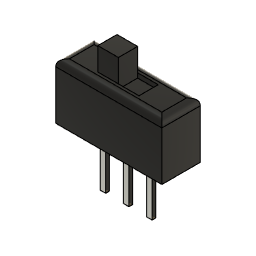
dropEgg_02 v12 (Autodesk Fusion 360 archive; units mm, degrees)
design "Switch"
Autodesk Fusion 360 part; units mm, degrees
sketch "Sketch1" plane through (0, 0, 0) normal (0, 0, 1) x (1, 0, 0)
  line L0 (5.8, -2.1) -> (-5.8, -2.1)
  line L1 (-5.8, -2.1) -> (-5.8, 2.1)
  line L2 (-5.8, 2.1) -> (5.8, 2.1)
  line L3 (5.8, 2.1) -> (5.8, -2.1)
  line L4 (5.8, -2.1) -> (-5.8, 2.1) construction
  line L5 (-5.8, -2.1) -> (5.8, 2.1) construction
  dimension "d1" = 11.6
  dimension "d2" = 4.2
  constraint horizontal L0
  constraint perpendicular L0 L1
  constraint parallel L0 L2
  constraint parallel L1 L3
  constraint coincident L4 origin
  constraint coincident L5 origin
  measures "d1" distance of L1.end L2.end
  measures "d2" distance of L0.end L1.end
extrude "Extrude1" add sketch "Sketch1" along normal blind 6.1
sketch "Sketch2" plane through (0, 0, 6.1) normal (0, 0, 1) x (-1, 0, 0)
  line L0 (-5.8, -2.1) -> (5.8, -2.1)
  line L1 (5.8, -2.1) -> (5.8, 2.1)
  line L2 (5.8, 2.1) -> (-5.8, 2.1)
  line L3 (-5.8, 2.1) -> (-5.8, -2.1)
  line L4 (-2.25, 1.05) -> (2.25, 1.05)
  line L5 (2.25, 1.05) -> (2.25, -1.05)
  line L6 (2.25, -1.05) -> (-2.25, -1.05)
  line L7 (-2.25, -1.05) -> (-2.25, 1.05)
  line L8 (-2.25, 1.05) -> (2.25, -1.05) construction
  line L9 (2.25, 1.05) -> (-2.25, -1.05) construction
  line L10 (0, -1.05) -> (0, 1.05)
  dimension "d5" = 4.5
  dimension "d6" = 2.1
  constraint horizontal L4
  constraint perpendicular L4 L5
  constraint parallel L4 L6
  constraint parallel L5 L7
  constraint coincident L8 origin
  constraint coincident L9 origin
  constraint midpoint L6 L10.start
  constraint midpoint L4 L10.end
  measures "d5" distance of L5.end L6.end
  measures "d6" distance of L4.end L5.end
extrude "Extrude2" add sketch "Sketch2" along normal blind 2.5 contours L4 L5 L6 L10
extrude "Extrude3" cut sketch "Sketch2" against normal blind 0.5 contours L4 L6 L7 L10
sketch "Sketch3" plane through (0, 0, 0) normal (0, 0, -1) x (1, 0, 0)
  line L0 (-5.8, -2.1) -> (5.8, -2.1)
  line L1 (5.8, -2.1) -> (5.8, 2.1)
  line L2 (5.8, 2.1) -> (-5.8, 2.1)
  line L3 (-5.8, 2.1) -> (-5.8, -2.1)
  line L4 (0.3, -0.2) -> (-0.3, -0.2)
  line L5 (-0.3, -0.2) -> (-0.3, 0.2)
  line L6 (-0.3, 0.2) -> (0.3, 0.2)
  line L7 (0.3, 0.2) -> (0.3, -0.2)
  line L8 (0.3, -0.2) -> (-0.3, 0.2) construction
  line L9 (-0.3, -0.2) -> (0.3, 0.2) construction
  dimension "d11" = 0.6
  dimension "d12" = 0.4
  constraint horizontal L4
  constraint perpendicular L4 L5
  constraint parallel L4 L6
  constraint parallel L5 L7
  constraint coincident L8 origin
  constraint coincident L9 origin
  measures "d11" distance of L5.end L6.end
  measures "d12" distance of L4.end L5.end
extrude "Extrude4" add sketch "Sketch3" along normal blind 5.8 contours L4 L5 L6 L7
pattern_linear "R-Pattern1" count 3 spacing 2.54 along (-1, 0, 0) both ways of "Extrude4"
fillet "Fillet1" radius 0.75 tangency weight 1.40143 4 edges at (-5.8, 0, 6.1) (5.8, 0, 6.1) (0, -2.1, 6.1) (0, 2.1, 6.1)

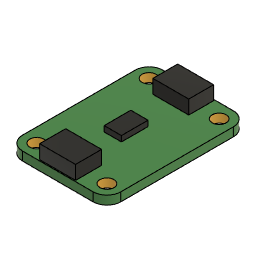
design "ADXL575"
Autodesk Fusion 360 part; units mm, degrees
sketch "Sketch1" plane through (0, 0, 0) normal (0, 0, 1) x (1, 0, 0)
  line L0 (8.89, -12.7) -> (-8.89, -12.7)
  line L1 (-8.89, -12.7) -> (-8.89, 12.7)
  line L2 (-8.89, 12.7) -> (8.89, 12.7)
  line L3 (8.89, 12.7) -> (8.89, -12.7)
  line L4 (8.89, -12.7) -> (-8.89, 12.7) construction
  line L5 (-8.89, -12.7) -> (8.89, 12.7) construction
  line L6 (6.35, -10.16) -> (-6.35, -10.16) construction
  line L7 (-6.35, -10.16) -> (-6.35, 10.16) construction
  line L8 (-6.35, 10.16) -> (6.35, 10.16) construction
  line L9 (6.35, 10.16) -> (6.35, -10.16) construction
  line L10 (6.35, -10.16) -> (-6.35, 10.16) construction
  line L11 (-6.35, -10.16) -> (6.35, 10.16) construction
  circle A0 centre (-6.35, 10.16) radius 1.27
  circle A1 centre (6.35, 10.16) radius 1.27
  circle A2 centre (-6.35, -10.16) radius 1.27
  circle A3 centre (6.35, -10.16) radius 1.27
  dimension "d1" = 17.78
  dimension "d2" = 25.4
  dimension "d3" = 12.7
  dimension "d4" = 20.32
  dimension "d5" = 2.54
  dimension "d6" = 2.54
  dimension "d7" = 2.54
  dimension "d8" = 2.54
  constraint horizontal L0
  constraint perpendicular L0 L1
  constraint parallel L0 L2
  constraint parallel L1 L3
  constraint coincident L4 origin
  constraint coincident L5 origin
  constraint horizontal L6
  constraint perpendicular L6 L7
  constraint parallel L6 L8
  constraint parallel L7 L9
  constraint coincident L10 origin
  constraint coincident L11 origin
  constraint coincident L7.end L8.start
  constraint coincident L8.end L9.start
  constraint coincident L6.end L7.start
  constraint coincident L6.start L9.end
  measures "d1" distance of L1.end L2.end
  measures "d2" distance of L0.end L1.end
  measures "d3" distance of L7.end L8.end
  measures "d4" distance of L6.end L7.end
  measures "d5" diameter of A0
  measures "d6" diameter of A1
  measures "d7" diameter of A2
  measures "d8" diameter of A3
extrude "Extrude1" add sketch "Sketch1" along normal blind 1.57
fillet "Fillet1" radius 2.5 4 edges at (-8.89, -12.7, 0.785) (8.89, -12.7, 0.785) (8.89, 12.7, 0.785) (-8.89, 12.7, 0.785)
sketch "Sketch2" plane through (0, 0, 1.57) normal (0, 0, 1) x (-1, 0, 0)
  arc A0 (6.39, -12.7) -> (8.89, -10.2) centre (6.39, -10.2) ccw
  line L0 (8.89, -10.2) -> (8.89, 10.2)
  arc A1 (8.89, 10.2) -> (6.39, 12.7) centre (6.39, 10.2) ccw
  line L1 (6.39, 12.7) -> (-6.39, 12.7)
  arc A2 (-6.39, 12.7) -> (-8.89, 10.2) centre (-6.39, 10.2) ccw
  line L2 (-8.89, 10.2) -> (-8.89, -10.2)
  arc A3 (-8.89, -10.2) -> (-6.39, -12.7) centre (-6.39, -10.2) ccw
  line L3 (-6.39, -12.7) -> (6.39, -12.7)
  circle A4 centre (6.35, -10.16) radius 1.27
  circle A5 centre (6.35, 10.16) radius 1.27
  circle A6 centre (-6.35, -10.16) radius 1.27
  circle A7 centre (-6.35, 10.16) radius 1.27
  line L4 (2, -2.5) -> (-1.1251, -2.5)
  line L5 (-1.1251, -2.5) -> (-1.1251, 2.3163)
  line L6 (-1.1251, 2.3163) -> (2, 2.3163)
  line L7 (2, 2.3163) -> (2, -2.5)
  line L8 (3.5, -12.5) -> (-3, -12.5)
  line L9 (-3, -12.5) -> (-3, -8)
  line L10 (-3, -8) -> (3.5, -8)
  line L11 (3.5, -8) -> (3.5, -12.5)
  line L12 (3.5, 12.5) -> (-3, 12.5)
  line L13 (-3, 12.5) -> (-3, 7.7871)
  line L14 (-3, 7.7871) -> (3.5, 7.7871)
  line L15 (3.5, 7.7871) -> (3.5, 12.5)
  constraint horizontal L4
  constraint vertical L5
  constraint horizontal L6
  constraint vertical L7
  constraint horizontal L8
  constraint vertical L9
  constraint horizontal L10
  constraint vertical L11
  constraint horizontal L12
  constraint vertical L13
  constraint horizontal L14
  constraint vertical L15
extrude "Extrude2" add sketch "Sketch2" along normal blind 2.5 contours L8 L9 L10 L11 | L12 L13 L14 L15
extrude "Extrude3" add sketch "Sketch2" along normal blind 1 contours L4 L5 L6 L7
equation "d1 = ( 0.7 * 25.4 ) * 1 mm"
equation "d3 = ( 0.5 * 25.4 ) * 1 mm"
equation "d4 = ( 0.8 * 25.4 ) * 1 mm"

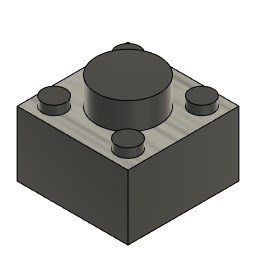
design "microswitch"
Autodesk Fusion 360 part; units mm, degrees
sketch "Sketch1" plane through (0, 0, 0) normal (0, 0, 1) x (1, 0, 0)
  line L0 (3.075, -3.075) -> (-3.075, -3.075)
  line L1 (-3.075, -3.075) -> (-3.075, 3.075)
  line L2 (-3.075, 3.075) -> (3.075, 3.075)
  line L3 (3.075, 3.075) -> (3.075, -3.075)
  line L4 (3.075, -3.075) -> (-3.075, 3.075) construction
  line L5 (-3.075, -3.075) -> (3.075, 3.075) construction
  circle A0 centre (0, 0) radius 1.75
  line L6 (2.05, 2.05) -> (-2.05, 2.05) construction
  line L7 (-2.05, 2.05) -> (-2.05, -2.05) construction
  line L8 (-2.05, -2.05) -> (2.05, -2.05) construction
  line L9 (2.05, -2.05) -> (2.05, 2.05) construction
  line L10 (2.05, 2.05) -> (-2.05, -2.05) construction
  line L11 (-2.05, 2.05) -> (2.05, -2.05) construction
  circle A1 centre (2.05, 2.05) radius 0.65
  circle A2 centre (-2.05, 2.05) radius 0.65
  circle A3 centre (-2.05, -2.05) radius 0.65
  circle A4 centre (2.05, -2.05) radius 0.65
  dimension "d1" = 6.15
  dimension "d2" = 6.15
  dimension "d3" = 3.5
  dimension "d8" = 1.3
  dimension "d9" = 4.1
  constraint horizontal L0
  constraint perpendicular L0 L1
  constraint parallel L0 L2
  constraint parallel L1 L3
  constraint coincident L4 A0.centre
  constraint coincident L5 A0.centre
  constraint coincident A0.centre origin
  constraint horizontal L6
  constraint perpendicular L6 L7
  constraint parallel L6 L8
  constraint parallel L7 L9
  constraint coincident L10 A0.centre
  constraint coincident L11 A0.centre
  constraint coincident L5 L6.start
  constraint coincident L6.start L9.end
  constraint coincident L6.end L7.start
  constraint coincident L7.end L8.start
  constraint coincident L8.end L9.start
  constraint equal A1 A4
  constraint equal A3 A4
  constraint equal A2 A3
  measures "d1" distance of L1.end L2.end
  measures "d2" distance of L0.end L1.end
  measures "d3" diameter of A0
  measures "d8" diameter of A1
  measures "d9" distance of L6.start L6.end
extrude "Extrude1" add sketch "Sketch1" against normal blind 3.6 contours L0 L1 L2 L3 | A0 | A1 | A2 | A3 | A4
extrude "Extrude2" add sketch "Sketch1" along normal blind 1.5 contours A0
extrude "Extrude3" add sketch "Sketch1" along normal blind 0.5 contours A1 | A2 | A3 | A4

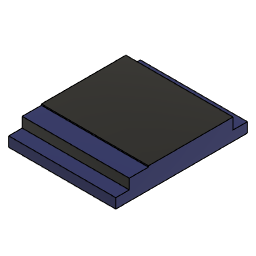
design "066_display"
Autodesk Fusion 360 part; units mm, degrees
sketch "Sketch1" plane through (0, 0, 0) normal (0, 0, 1) x (1, 0, 0)
  line L0 (9.5, 11.675) -> (-9.5, 11.675)
  line L1 (-9.5, 11.675) -> (-9.5, -11.675)
  line L2 (-9.5, -11.675) -> (9.5, -11.675)
  line L3 (9.5, -11.675) -> (9.5, 11.675)
  line L4 (9.5, 11.675) -> (-9.5, -11.675) construction
  line L5 (-9.5, 11.675) -> (9.5, -11.675) construction
  circle A0 centre (-3.81, 10.375) radius 0.45
  dimension "d1" = 19
  dimension "d2" = 23.35
  dimension "d9" = 0.9
  dimension "d10" = 1.3
  dimension "d11" = 3.81
  constraint horizontal L0
  constraint perpendicular L0 L1
  constraint parallel L0 L2
  constraint parallel L1 L3
  constraint coincident L4 origin
  constraint coincident L5 origin
  measures "d1" distance of L1.end L2.end
  measures "d2" distance of L0.end L1.end
  measures "d9" diameter of A0
  measures "d10" distance of L0 A0.centre
  measures "d11" horizontal distance of origin A0.centre
extrude "Extrude1" add sketch "Sketch1" along normal blind 1.75
sketch "Sketch2" plane through (0, 0, 1.75) normal (0, 0, 1) x (-1, 0, 0)
  line L0 (-9.5, 11.675) -> (-9.5, -11.675)
  line L1 (-9.5, -11.675) -> (9.5, -11.675)
  line L2 (9.5, -11.675) -> (9.5, 11.675)
  line L3 (9.5, 11.675) -> (-9.5, 11.675)
  line L4 (9.5, -9.125) -> (-9.5, -9.125)
  line L5 (-9.5, -9.125) -> (-9.5, 9.275)
  line L6 (-9.5, 9.275) -> (9.5, 9.275)
  line L7 (9.5, 9.275) -> (9.5, -9.125)
  circle A0 centre (3.81, -10.375) radius 0.45
  dimension "d5" = 2.55
  dimension "d6" = 2.4
  constraint horizontal L4
  constraint vertical L5
  constraint horizontal L6
  constraint vertical L7
  constraint coincident L0 L5.end
  constraint coincident L2 L4.start
  measures "d5" distance of L1 L4
  measures "d6" distance of L3 L6
extrude "Extrude2" add sketch "Sketch2" along normal blind 2 contours L0 L2 L4 L5 L6 L7
pattern_linear "R-Pattern1" count 4 spacing 2.54 along (1, 0, 0) of 1 faces at (-3.3689, 10.2858, 1.1667)
sketch "Sketch3" plane through (0, 0, 3.75) normal (0, 0, 1) x (-1, 0, 0)
  line L0 (9.5, 9.275) -> (-9.5, 9.275)
  line L1 (-9.5, 9.275) -> (-9.5, -9.125)
  line L2 (-9.5, -9.125) -> (9.5, -9.125)
  line L3 (9.5, -9.125) -> (9.5, 9.275)
  line L4 (9.5, -9.125) -> (-9.5, -9.125)
  line L5 (-9.5, -9.125) -> (-9.5, 5.875)
  line L6 (-9.5, 5.875) -> (9.5, 5.875)
  line L7 (9.5, 5.875) -> (9.5, -9.125)
  dimension "d16" = 15
  constraint horizontal L4
  constraint vertical L5
  constraint horizontal L6
  constraint vertical L7
  constraint coincident L1 L5.end
  constraint coincident L2.end L3.start
  measures "d16" distance of L4 L6
extrude "Extrude3" cut sketch "Sketch3" against normal blind 0.2 contours L0 L1 L3 L6
equation "d11 = ( 0.15 * 25.4 ) * 1 mm"

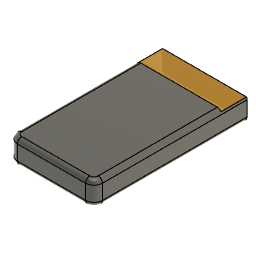
design "LiPo"
Autodesk Fusion 360 part; units mm, degrees
sketch "Sketch1" plane through (0, 0, 0) normal (0, 0, 1) x (1, 0, 0)
  line L0 (10, 18) -> (-10, 18)
  line L1 (-10, 18) -> (-10, -18)
  line L2 (-10, -18) -> (10, -18)
  line L3 (10, -18) -> (10, 18)
  line L4 (10, 18) -> (-10, -18) construction
  line L5 (-10, 18) -> (10, -18) construction
  dimension "d1" = 20
  dimension "d2" = 36
  constraint horizontal L0
  constraint perpendicular L0 L1
  constraint parallel L0 L2
  constraint parallel L1 L3
  constraint coincident L4 origin
  constraint coincident L5 origin
  measures "d1" distance of L1.end L2.end
  measures "d2" distance of L0.end L1.end
extrude "Extrude1" add sketch "Sketch1" along normal blind 5.5
sketch "Sketch2" plane through (0, 0, 5.5) normal (0, 0, 1) x (-1, 0, 0)
  line L0 (-10, 18) -> (-10, -18)
  line L1 (-10, -18) -> (10, -18)
  line L2 (10, -18) -> (10, 18)
  line L3 (10, 18) -> (-10, 18)
  line L4 (10, -18) -> (-10.3, -18)
  line L5 (-10.3, -18) -> (-10.3, -12)
  line L6 (-10.3, -12) -> (10, -12)
  line L7 (10, -12) -> (10, -18)
  dimension "d5" = 20.3
  dimension "d6" = 6
  constraint horizontal L4
  constraint vertical L5
  constraint horizontal L6
  constraint vertical L7
  constraint coincident L1.end L2.start
  measures "d5" distance of L1.end L4.end
  measures "d6" distance of L1.end L6.end
extrude "Extrude2" cut sketch "Sketch2" against normal blind 0.5 contours L0 L1 L2 L4 L6 L7 | L0 L4 L5 L6
fillet "Fillet1" radius 2 2 edges at (-10, -18, 2.75) (10, -18, 2.75)
fillet "Fillet2" radius 1 10 edges at (-10, -2, 5.5) (-9.4142, -17.4142, 5.5) (0, -18, 5.5) (9.4142, -17.4142, 5.5) (10, -2, 5.5) (-10, 1, 0) (-9.4142, -17.4142, 0) (0, -18, 0) (9.4142, -17.4142, 0) (10, 1, 0)
